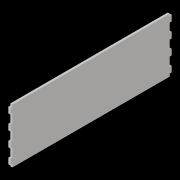
# Autodesk Inventor part: Back V3
Saved by Autodesk Inventor 2018 (Build 220112000, 112)
## iProperties
Created: 2017-09-13
Part Number: Back V3
Material: Generic
Document SubType Name: Modeling
Designer: gaine
Density: 1 g/cm^3
Appearance: Default
Author: gaine
Autodesk Inventor part; units mm, degrees
ref_plane "YZ Plane" through (0, 0, 0) normal (1, 0, 0) x (0, 1, 0)
ref_plane "XZ Plane" through (0, 0, 0) normal (0, 1, 0) x (-1, 0, 0)
ref_plane "XY Plane" through (0, 0, 0) normal (0, 0, 1) x (1, 0, 0)
sketch "Sketch1" plane through (0, 0, 0) normal (1, 0, 0) x (0, 1, 0)
  line L0 (-177.971, 517.5894) -> (-177.971, -12.6356)
  line L1 (5.0614, -12.6356) -> (5.0614, 517.5894)
  line L2 (-1.2886, 523.9394) -> (-20.3386, 523.9394)
  line L3 (-20.3386, 523.9394) -> (-20.3386, 517.5894)
  line L4 (-1.2886, 517.5894) -> (-1.2886, 523.9394)
  line L5 (-50.8186, 523.9394) -> (-69.8686, 523.9394)
  line L6 (-69.8686, 523.9394) -> (-69.8686, 517.5894)
  line L7 (-50.8186, 517.5894) -> (-50.8186, 523.9394)
  line L8 (-100.3486, 523.9394) -> (-119.3986, 523.9394)
  line L9 (-119.3986, 523.9394) -> (-119.3986, 517.5894)
  line L10 (-100.3486, 517.5894) -> (-100.3486, 523.9394)
  line L11 (-168.9286, 523.9394) -> (-149.8786, 523.9394)
  line L12 (-149.8786, 523.9394) -> (-149.8786, 517.5894)
  line L13 (-168.9286, 517.5894) -> (-168.9286, 523.9394)
  line L14 (-168.9286, 517.5894) -> (-177.971, 517.5894)
  line L15 (-149.8786, 517.5894) -> (-119.3986, 517.5894)
  line L16 (-100.3486, 517.5894) -> (-69.8686, 517.5894)
  line L17 (-50.8186, 517.5894) -> (-20.3386, 517.5894)
  line L18 (-1.2886, 517.5894) -> (5.0614, 517.5894)
  line L19 (-149.8786, 523.9394) -> (-168.9286, 523.9394)
  line L20 (-100.3486, 523.9394) -> (-119.3986, 523.9394)
  line L21 (-1.2886, 523.9394) -> (-20.3386, 523.9394)
  line L22 (-50.8186, 523.9394) -> (-69.8686, 523.9394)
  line L23 (-1.2886, -18.9856) -> (-1.2886, -12.6356)
  line L24 (-1.2886, -12.6356) -> (5.0614, -12.6356)
  line L25 (-50.8186, -18.9856) -> (-50.8186, -12.6356)
  line L26 (-50.8186, -12.6356) -> (-20.3386, -12.6356)
  line L27 (-20.3386, -12.6356) -> (-20.3386, -18.9856)
  line L28 (-100.3486, -18.9856) -> (-100.3486, -12.6356)
  line L29 (-100.3486, -12.6356) -> (-69.8686, -12.6356)
  line L30 (-69.8686, -12.6356) -> (-69.8686, -18.9856)
  line L31 (-149.8786, -18.9856) -> (-149.8786, -12.6356)
  line L32 (-149.8786, -12.6356) -> (-119.3986, -12.6356)
  line L33 (-119.3986, -12.6356) -> (-119.3986, -18.9856)
  line L34 (-168.9286, -18.9856) -> (-168.9286, -12.6356)
  line L35 (-168.9286, -12.6356) -> (-177.971, -12.6356)
  line L36 (-168.9286, -18.9856) -> (-149.8786, -18.9856)
  line L37 (-119.3986, -18.9856) -> (-100.3486, -18.9856)
  line L38 (-69.8686, -18.9856) -> (-50.8186, -18.9856)
  line L39 (-20.3386, -18.9856) -> (-1.2886, -18.9856)
  point P0 (0, 0)
  dimension "d15" = 6.35
  dimension "d16" = 6.35
  dimension "d17" = 19.05
  dimension "d18" = 30.48
  dimension "d19" = 6.35
  dimension "d20" = 19.05
  dimension "d21" = 6.35
  dimension "d22" = 30.48
  dimension "d23" = 19.05
  dimension "d24" = 30.48
  dimension "d25" = 6.35
  dimension "d26" = 19.05
  dimension "d27" = 9.0424
  dimension "d43" = 542.925
  dimension "d44" = 183.0324
  dimension "d45" = 19.05
  dimension "d46" = 30.48
  dimension "d47" = 19.05
  dimension "d48" = 30.48
  dimension "d49" = 19.05
  dimension "d50" = 30.48
  dimension "d51" = 19.05
  dimension "d52" = 9.0424
  dimension "d53" = 6.35
  dimension "d54" = 6.35
  dimension "d55" = 6.35
  dimension "d56" = 6.35
  dimension "d57" = 6.35
  constraints: 80 end point, 24 parallel, 9 perpendicular, 8 horizontal, 7 collinear, 1 point on line
  measures "d15" distance between parallel lines of L4 L1
  measures "d16" distance between parallel lines of L18 L2
  measures "d17" distance between parallel lines of L3 L4
  measures "d18" distance between parallel lines of L7 L3
  measures "d19" distance between parallel lines of L17 L5
  measures "d20" distance between parallel lines of L6 L7
  measures "d21" distance between parallel lines of L16 L8
  measures "d22" distance between parallel lines of L10 L6
  measures "d23" distance between parallel lines of L9 L10
  measures "d24" distance between parallel lines of L12 L9
  measures "d25" distance between parallel lines of L15 L11
  measures "d26" distance between parallel lines of L13 L12
  measures "d27" distance between parallel lines of L0 L13
  measures "d43" distance between parallel lines of L2 L39
  measures "d44" distance between parallel lines of L0 L1
  measures "d45" distance between parallel lines of L27 L23
  measures "d46" distance between parallel lines of L25 L27
  measures "d47" distance between parallel lines of L30 L25
  measures "d48" distance between parallel lines of L28 L30
  measures "d49" distance between parallel lines of L33 L28
  measures "d50" distance between parallel lines of L31 L33
  measures "d51" distance between parallel lines of L34 L31
  measures "d52" distance between parallel lines of L0 L34
  measures "d53" distance between parallel lines of L23 L1
  measures "d54" distance between parallel lines of L39 L24
  measures "d55" distance between parallel lines of L38 L26
  measures "d56" distance between parallel lines of L37 L29
  measures "d57" distance between parallel lines of L36 L32
extrude "Extrusion1" add sketch "Sketch1" along normal blind 6.35
body "Solid1"
